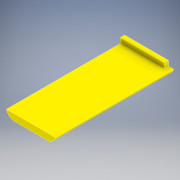
# Autodesk Inventor part: Case_Cover
Saved by Autodesk Inventor 2020 (Build 240168000, 168)
## iProperties
Created: 2019-11-07
Part Number: Case_Cover
Material: 일반
Document SubType Name: Modeling
Designer: Knowblesse
Density: 1 g/cm^3
Appearance: 기본값
Author: Knowblesse
## iProperties of the stored document _3D 인쇄.ipt
Created: 2020-07-23
Part Number: _3D 인쇄
Material: 일반
Document SubType Name: Modeling
Designer: Knowblesse
Density: 1 g/cm^3
Appearance: 기본값
Author: Knowblesse
Autodesk Inventor part; units mm, degrees
ref_plane "YZ Plane" through (0, 0, 0) normal (1, 0, 0) x (0, 1, 0)
ref_plane "XZ Plane" through (0, 0, 0) normal (0, 1, 0) x (-1, 0, 0)
ref_plane "XY Plane" through (0, 0, 0) normal (0, 0, 1) x (1, 0, 0)
sketch "스케치1" plane through (0, 0, 0) normal (0, 1, 0) x (-1, 0, 0)
  line L0 (0, 0) -> (11.4, 0)
  line L1 (11.4, 0) -> (11.4, -27.5)
  line L2 (11.4, -27.5) -> (0, -27.5)
  line L3 (0, -27.5) -> (0, 0)
  dimension "d0" = 11.4
  dimension "d1" = 27.5
  constraints: 8 end point, 2 parallel, 1 horizontal, 1 perpendicular
  measures "d0" distance of L1.end L2.end
  measures "d1" distance of L0.end L1.end
extrude "돌출1" add sketch "스케치1" along normal blind 1.5
fillet "모깎기1" radius 2 2 edges at (-11.4, 0, -13.75) (0, 0, -13.75)
sketch "스케치4" plane through (0, 1.5, 0) normal (0, 1, 0) x (1, 0, 0)
  line L0 (-11.4, 27.5) -> (-11.4, 0) projected
  line L1 (0, 0) -> (0, 27.5) projected
  line L2 (0, 27.5) -> (-11.4, 27.5) projected
  line L3 (-11.4, 27.5) -> (0, 27.5)
  line L4 (0, 27.5) -> (0, 26.5)
  line L5 (0, 26.5) -> (-11.4, 26.5)
  line L6 (-11.4, 26.5) -> (-11.4, 27.5)
  line L7 (-1.2, 26.5) -> (-1.2, 27.5)
  dimension "d18" = 1
  dimension "d21" = 1.2
  constraints: 10 end point, 3 point on line, 2 parallel, 2 perpendicular, 1 horizontal
  measures "d18" distance of L3.end L4.end
  measures "d21" distance between parallel lines of L7 L1
extrude "돌출4" add sketch "스케치4" along normal blind 1.2 contours L2 L7 L5 L0
